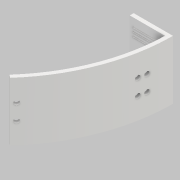
# Autodesk Inventor part: CW002
Saved by Autodesk Inventor 2017 (Build 210142000, 142)
## iProperties
Created: 2017-05-22
Part Number: CW002
Material: ABS Plastic
Document SubType Name: Modeling
Designer: zallen
Density: 1.06 g/cm^3
Appearance: CR White
Author: zallen
Autodesk Inventor part; units mm, degrees
ref_plane "YZ Plane" through (0, 0, 0) normal (1, 0, 0) x (0, 1, 0)
ref_plane "XZ Plane" through (0, 0, 0) normal (0, 1, 0) x (-1, 0, 0)
ref_plane "XY Plane" through (0, 0, 0) normal (0, 0, 1) x (1, 0, 0)
sketch "Sketch1" plane through (0, 0, 0) normal (0, 0, 1) x (1, 0, 0)
  line L0 (0, 0) -> (50, 0)
  line L1 (50, 0) -> (50, 5)
  line L2 (50, 5) -> (0, 5)
  line L3 (0, 5) -> (0, 0)
  dimension "d0" = 50
  dimension "d1" = 5
  constraints: 8 end point, 2 parallel, 1 horizontal, 1 perpendicular
  measures "d0" distance of L2.end L1.end
  measures "d1" distance of L1.end L0.end
extrude "Extrusion1" add sketch "Sketch1" along normal blind 75
sketch "Sketch2" plane through (0, 0, 0) normal (-1, 0, 0) x (0, 0, 1)
  circle A0 centre (47.5, 2.5) radius 1
  circle A1 centre (27.5, 2.5) radius 1
  line L0 (0, 5) -> (0, 0) projected
  line L1 (0, 0) -> (75, 0) projected
  dimension "d4" = 2
  dimension "d5" = 2
  dimension "d6" = 27.5
  dimension "d7" = 20
  dimension "d8" = 2.5
  constraints: 2 centre point, 1 horizontal alignment
  measures "d4" diameter of A0
  measures "d5" diameter of A1
  measures "d6" distance from line of L0 A1.centre
  measures "d7" distance of A1.centre A0.centre
  measures "d8" distance from line of L1 A1.centre
extrude "Extrusion2" cut sketch "Sketch2" against normal blind 10
thread "Thread1" size "M2x0.4" class "6H" standard "ANSI Metric M Profile" full length
thread "Thread2" size "M2x0.4" class "6H" standard "ANSI Metric M Profile" full length
sketch "Sketch6" plane through (0, 0, 0) normal (0, 0, 1) x (1, 0, 0)
  circle A0 centre (-175, 5) radius 225 construction
  line L0 (-7.3973, 5.2329) -> (-7.3973, -145.1144) construction
  line L1 (-176.0104, 5) -> (50, 5) construction
  circle A1 centre (-175, 5) radius 220 construction
  arc A2 (-7.3973, -145.1144) -> (50, 5) centre (-175, 5) ccw
  line L2 (-7.3973, -145.1144) -> (-11.1218, -141.7785)
  arc A3 (-11.1218, -141.7785) -> (45, 5) centre (-175, 5) ccw
  line L3 (0, 5) -> (50, 5)
  line L4 (45, 5) -> (50, 5)
  point P0 (0, 5)
  dimension "d2" = 75
  dimension "d36" = 450
  dimension "d38" = 5
  dimension "d39" = 5
  dimension "d69" = 150.1144
  constraints: 10 end point, 9 point on circle, 4 centre point, 2 concentric, 2 horizontal alignment, 1 coincident, 1 horizontal, 1 point on line, 1 vertical
  measures "d36" diameter of A0
  measures "d38" radial gap between concentric circles of A0 A1
  measures "d39" distance of L0.end L2.end
  measures "d69" vertical distance of point (50, 5) L0.end
extrude "Extrusion5" add sketch "Sketch6" along normal blind 75
ref_plane "Work Plane3" through (50, 2.5, 0) normal (-0.9319544, 0.3623741, 0.0120791) x (-0.3624006, -0.9320224, 0)
sketch "Sketch7" plane through (50, 2.5, 0) normal (-0.9319544, 0.3623741, 0.0120791) x (-0.3624006, -0.9320224, 0)
  circle A0 centre (27.1699, 27.4836) radius 3
  circle A1 centre (27.1699, 47.4836) radius 3
  line L0 (-2.3301, -0.0109) -> (-2.3301, 74.9836) projected
  circle A2 centre (37.1699, 27.4836) radius 3
  circle A3 centre (37.1699, 47.4836) radius 3
  point P0 (20.4501, -0.552)
  dimension "d42" = 6
  dimension "d43" = 6
  dimension "d44" = 29.5
  dimension "d46" = 20
  dimension "d47" = 27.5
  dimension "d48" = 6
  dimension "d49" = 6
  dimension "d50" = 10
  constraints: 4 centre point, 2 horizontal alignment, 2 vertical alignment
  measures "d42" diameter of A0
  measures "d43" diameter of A1
  measures "d44" distance from line of A0.centre L0
  measures "d46" distance of A0.centre A1.centre
  measures "d47" vertical distance of L0.end A1.centre
  measures "d48" diameter of A2
  measures "d49" diameter of A3
  measures "d50" distance of A2.centre A0.centre
extrude "Extrusion6" cut sketch "Sketch7" along normal through all both and the other way through all
sketch "Sketch8" plane through (0, 5, 0) normal (0, 1, 0) x (1, 0, 0)
  line L0 (3.75, -65) -> (46.25, -65)
  line L1 (46.25, -65) -> (46.25, -63)
  line L2 (46.25, -63) -> (3.75, -63)
  line L3 (3.75, -63) -> (3.75, -65)
  line L4 (50, 0) -> (0, 0) projected
  line L5 (0, 0) -> (0, -75) projected
  line L6 (50, -75) -> (0, -75) projected
  line L7 (50, 0) -> (50, -75) projected
  line L8 (46.25, -58) -> (3.75, -58)
  line L9 (3.75, -58) -> (3.75, -60)
  line L10 (3.75, -60) -> (46.25, -60)
  line L11 (46.25, -60) -> (46.25, -58)
  line L12 (46.25, -53) -> (3.75, -53)
  line L13 (3.75, -53) -> (3.75, -55)
  line L14 (3.75, -55) -> (46.25, -55)
  line L15 (46.25, -55) -> (46.25, -53)
  dimension "d56" = 42.5
  dimension "d57" = 2
  dimension "d58" = 3.75
  dimension "d59" = 10
  dimension "d62" = 5
  constraints: 24 end point, 2 parallel, 1 horizontal, 1 perpendicular, 1 vertical, 16 other
  measures "d56" distance of L2.end L1.end
  measures "d57" distance of L0.end L1.end
  measures "d58" horizontal distance of point (0, -75) L0.start
  measures "d59" vertical distance of L6.start L0.end
  measures "d62" distance of L1.end L8.start
extrude "Extrusion7" cut sketch "Sketch8" against normal blind 5 contours L3 L2 L1 L0 | L11 L10 L9 L8 | L15 L14 L13 L12
ref_plane "Work Plane4" through (-7.3973, -145.1144, 0) normal (0.7449011, -0.6671749, 0) x (0.6671749, 0.7449011, 0)
sketch "Sketch9" plane through (-7.3973, -145.1144, 0) normal (0.7449011, -0.6671749, 0) x (0.6671749, 0.7449011, 0)
  circle A0 centre (6, 27.5) radius 3
  circle A1 centre (6, 47.5) radius 3
  line L0 (146.3528, 75) -> (0, 75) projected
  line L1 (0, 0) -> (0, 75) projected
  point P0 (113.0311, 0)
  dimension "d70" = 6
  dimension "d71" = 6
  dimension "d72" = 27.5
  dimension "d73" = 20
  dimension "d74" = 6
  constraints: 2 centre point, 1 vertical alignment
  measures "d70" diameter of A0
  measures "d71" diameter of A1
  measures "d72" distance from line of L0 A1.centre
  measures "d73" distance of A0.centre A1.centre
  measures "d74" distance from line of A1.centre L1
extrude "Extrusion8" cut sketch "Sketch9" along normal through all both and the other way through all
body "Solid1"
